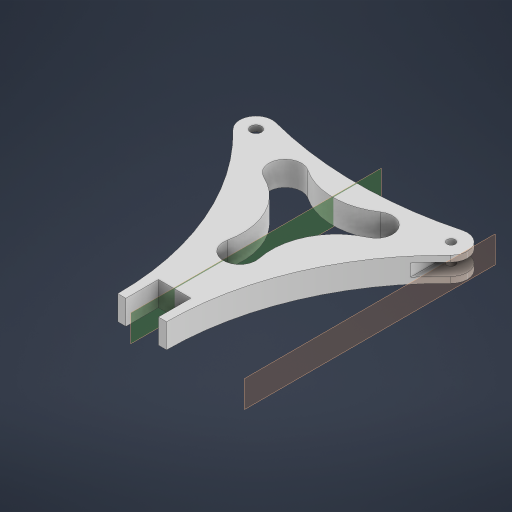
# Autodesk Inventor part: shock_absorber_holder
Saved by Autodesk Inventor 2024 (Build 280153000, 153)
## iProperties
Created: 2023-05-05
Part Number: shock_absorber_holder
Material: Типовые
Document SubType Name: Modeling
Designer: user
Density: 1 g/cm^3
Appearance: По умолчанию
Mass: 95.4109 g
Surface Area: 248.354 cm^2
Volume: 95.4109 cm^3
Author: user
Autodesk Inventor part; units mm, degrees
ref_plane "YZ Plane" through (0, 0, 0) normal (1, 0, 0) x (0, 1, 0)
ref_plane "XZ Plane" through (0, 0, 0) normal (0, 1, 0) x (-1, 0, 0)
ref_plane "XY Plane" through (0, 0, 0) normal (0, 0, 1) x (1, 0, 0)
sketch "Эскиз1" plane through (0, 0, 0) normal (0, 0, 1) x (1, 0, 0)
  line L0 (20, 0) -> (20, 20)
  line L1 (20, 20) -> (0, 20)
  line L2 (0, 20) -> (0, 0)
  arc A0 (-47.4468, 139.6686) -> (-56.9636, 122.8231) centre (-50, 130) ccw
  arc A1 (76.9636, 122.8231) -> (67.4468, 139.6686) centre (70, 130) ccw
  arc A2 (-47.4468, 139.6686) -> (67.4468, 139.6686) centre (10, 357.2114) ccw
  line L3 (0, 0) -> (-5, 0)
  line L4 (20, 0) -> (25, 0)
  arc A3 (-5, 0) -> (-56.9636, 122.8231) centre (-176.1364, 0) ccw
  arc A4 (76.9636, 122.8231) -> (25, 0) centre (196.1364, 0) ccw
  arc A5 (42.1742, 106.9129) -> (19.7742, 62.1129) centre (58.8712, 70.5644) ccw
  arc A6 (42.1742, 106.9129) -> (32.4, 124.2849) centre (38, 116) ccw
  arc A7 (-12.4, 124.2849) -> (32.4, 124.2849) centre (10, 157.4246) ccw
  arc A8 (-12.4, 124.2849) -> (-22.1742, 106.9129) centre (-18, 116) ccw
  arc A9 (0.2258, 62.1129) -> (-22.1742, 106.9129) centre (-38.8712, 70.5644) ccw
  arc A10 (0.2258, 62.1129) -> (19.7742, 62.1129) centre (10, 60) ccw
  circle A11 centre (-50, 130) radius 3.3777
  circle A12 centre (70, 130) radius 2.5532
  point P0 (10, 181.6134)
  point P1 (10, 20)
  point P2 (10, 132.2114)
  point P3 (10, 117.4246)
  dimension "d0" = 20
  dimension "d5" = 120
  dimension "d6" = 20
  dimension "d9" = 5
  dimension "d10" = 130
  dimension "d12" = 10
  dimension "d13" = 225
  dimension "d14" = 56
  dimension "d15" = 56
  dimension "d16" = 10
  dimension "d17" = 40
  dimension "d18" = 40
  constraints: 24 point on circle, 13 centre point, 10 end point, 9 tangent, 5 equal radius, 5 vertical alignment, 3 horizontal, 3 horizontal alignment, 2 coincident, 2 line through centre, 1 collinear, 1 midpoint, 1 parallel, 1 vertical
  measures "d0" distance of L0.start L2.end
  measures "d5" distance of A0.centre A1.centre
  measures "d6" distance of L0.start L0.end
  measures "d9" distance of L2.end L3.end
  measures "d10" vertical distance of L3.end A0.centre
  measures "d12" radius of A1
  measures "d13" radius of A2
  measures "d14" distance of A6.centre A8.centre
  measures "d15" vertical distance of A10.centre A8.centre
  measures "d16" radius of A10
  measures "d17" vertical distance of L1.end A10.centre
  measures "d18" radius of A5
extrude "Выдавливание1" add sketch "Эскиз1" along normal blind 15
ref_plane "РабПлоскость2" through (80, 130, 0) normal (1, 0, 0) x (0, 0, -1)
sketch "Эскиз3" plane through (80, 130, 0) normal (1, 0, 0) x (0, 0, -1)
  line L0 (0, 10) -> (-15, 10) projected
  line L1 (0, -7.1769) -> (-15, -7.1769) projected
  line L2 (-11.275, 10) -> (-3.725, 10)
  line L3 (-3.725, 10) -> (-3.725, -7.1769)
  line L4 (-3.725, -7.1769) -> (-11.275, -7.1769)
  line L5 (-11.275, -7.1769) -> (-11.275, 10)
  point P0 (0, -130)
  point P1 (-7.5, 10)
  point P2 (-7.5, 10)
  dimension "d23" = 7.55
  constraints: 8 end point, 2 midpoint, 2 parallel, 2 point on line, 1 coincident, 1 horizontal, 1 perpendicular
  measures "d23" distance of L2.end L2.start
extrude "Выдавливание3" cut sketch "Эскиз3" against normal blind 15
ref_plane "РабПлоскость4" through (10, 132.2114, 0) normal (-1, 0, 0) x (0, 0, 1)
move faces "Перенос1" translate (0, -22, 0) faces at (72.9757, 122.8231, 8.7583)
ref_plane "РабПлоскость3" through (10, 132.2114, 0) normal (-1, 0, 0) x (0, 0, 1)
mirror "Зеркальное отражение1" about plane through (10, 132.2114, 0) normal (-1, 0, 0) of "Выдавливание3"
move faces "Перенос2" translate (0, -26.5, 0) faces at (-52.9757, 122.8231, 8.7583)
